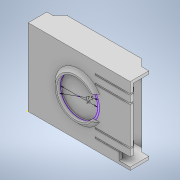
# Autodesk Inventor part: ButtonBatteryHolder
Saved by Autodesk Inventor 2022 (Build 260153000, 153)
## iProperties
Created: 2022-08-02
Part Number: ButtonBatteryHolder
Material: Generic
Document SubType Name: Modeling
Designer: sgioj
Density: 1 g/cm^3
Appearance: Default
Author: sgioj
Autodesk Inventor part; units mm, degrees
ref_plane "YZ Plane" through (0, 0, 0) normal (1, 0, 0) x (0, 1, 0)
ref_plane "XZ Plane" through (0, 0, 0) normal (0, 1, 0) x (-1, 0, 0)
ref_plane "XY Plane" through (0, 0, 0) normal (0, 0, 1) x (1, 0, 0)
sketch "Sketch1" plane through (0, 0, 0) normal (0, 0, 1) x (1, 0, 0)
  line L0 (0, 0) -> (44, 0)
  line L1 (44, 0) -> (44, 33)
  line L2 (44, 33) -> (0, 33)
  line L3 (0, 33) -> (0, 0)
  line L4 (2, 1.5) -> (44, 1.5)
  line L5 (44, 1.5) -> (44, 31.5)
  line L6 (44, 31.5) -> (2, 31.5)
  line L7 (2, 31.5) -> (2, 1.5)
  dimension "d0" = 44
  dimension "d1" = 33
  dimension "d2" = 42
  dimension "d3" = 30
  dimension "d4" = 2
  dimension "d5" = 0
  dimension "d6" = 1.5
  constraints: 16 end point, 4 parallel, 2 horizontal, 2 perpendicular
  measures "d0" distance of L2.end L1.end
  measures "d1" distance of L1.end L0.end
  measures "d2" distance of L6.end L5.end
  measures "d3" distance of L5.end L4.end
  measures "d4" distance between parallel lines of L7 L3
  measures "d5" distance between parallel lines of L1 L5
  measures "d6" distance between parallel lines of L4 L0
extrude "Extrusion1" add sketch "Sketch1" along normal blind 11
shell "Shell1" thickness 1.25 removed faces 1 at (44, 11, 3.6667)
sketch "Sketch2" plane through (0, 0, 11) normal (0, 0, 1) x (1, 0, 0)
  circle A0 centre (22, 16.5) radius 8
  circle A1 centre (22, 16.5) radius 8.75
  point P0 (0, 0)
  dimension "d10" = 16
  dimension "d11" = 17.5
  constraints: 2 centre point, 1 coincident
  measures "d10" diameter of A0
  measures "d11" diameter of A1
extrude "Extrusion2" add sketch "Sketch2" along normal blind 1.5
sketch "Sketch3" plane through (22, 16.5, 11) normal (0, 0, 1) x (1, 0, 0)
  line L0 (1.47, 5.1769) -> (11.6334, 5.1769)
  line L1 (11.6334, 5.1769) -> (11.6334, -5.2059)
  line L2 (11.6334, -5.2059) -> (1.47, -5.2059)
  line L3 (1.47, -5.2059) -> (1.47, 5.1769)
  line L4 (1.47, 5.1769) -> (11.6334, -5.2059) construction
  line L5 (11.6334, 5.1769) -> (1.47, -5.2059) construction
  point P0 (-22, -16.5)
  point P1 (6.5517, -0.0145)
  constraints: 12 end point, 2 midpoint, 2 parallel, 1 horizontal, 1 perpendicular
extrude "Extrusion3" cut sketch "Sketch2" against normal blind 0.6 contours A0
sketch "Sketch4" plane through (0, 0, 0) normal (0, 0, -1) x (-1, 0, 0)
  circle A0 centre (-22, 16.5) radius 8.7
  line L0 (-44, 33) -> (0, 33) projected
  line L1 (0, 33) -> (0, 0) projected
  dimension "d16" = 17.4
  dimension "d22" = 16.5
  dimension "d23" = 22
  constraints: 1 centre point
  measures "d16" diameter of A0
  measures "d22" distance from line of L0 A0.centre
  measures "d23" distance from line of L1 A0.centre
extrude "Extrusion4" cut sketch "Sketch4" against normal blind 0.6
chamfer "Chamfer1" distance 1.5 angle 45 1 edges at (13.25, 16.5, 11)
extrude "Extrusion5" cut sketch "Sketch3" along normal blind 2
sketch "Sketch5" plane through (0, 33, 0) normal (0, 1, 0) x (1, 0, 0)
  line L0 (0, 0) -> (3, 0)
  line L1 (3, 0) -> (3, -3)
  line L2 (3, -3) -> (0, -3)
  line L3 (0, -3) -> (0, 0)
  line L4 (0, 0) -> (44, 0) projected
  line L5 (44, 0) -> (41, 0)
  line L6 (41, 0) -> (41, -3)
  line L7 (41, -3) -> (44, -3)
  line L8 (44, -3) -> (44, 0)
  dimension "d26" = 3
  dimension "d27" = 3
  dimension "d28" = 3
  dimension "d29" = 3
  constraints: 16 end point, 4 parallel, 2 horizontal, 2 perpendicular
  measures "d26" distance of L1.end L2.end
  measures "d27" distance of L0.end L1.end
  measures "d28" distance of L7.end L6.end
  measures "d29" distance of L6.end L5.end
extrude "Extrusion6" cut sketch "Sketch5" against normal through all
sketch "Sketch6" plane through (0, 0, 11) normal (-1, 0, 0) x (0, 0, 1)
  line L0 (0, 0) -> (0, 33) projected
  line L1 (-11, 33) -> (-11, 0) projected
  line L2 (0, 0) -> (-11, 0)
  line L3 (-11, 0) -> (-11, 33)
  line L4 (-11, 33) -> (0, 33)
  line L5 (0, 33) -> (0, 0)
  constraints: 8 end point, 2 parallel, 1 horizontal, 1 perpendicular
extrude "Extrusion7" cut sketch "Sketch6" against normal blind 0.25
chamfer "Chamfer2" distance 3 angle 45 2 edges at (3, 16.5, 0) (41, 16.5, 0)
sketch "Sketch7" plane through (0, 0, 11) normal (0, 0, 1) x (1, 0, 0)
  line L0 (44, 1.25) -> (44, 31.75) projected
  line L1 (44, 28) -> (29, 28)
  line L2 (29, 28) -> (29, 25)
  line L3 (29, 25) -> (44, 25)
  line L4 (44, 25) -> (44, 28)
  line L5 (44, 33) -> (0.25, 33) projected
  line L6 (44, 28.5) -> (29, 28.5)
  line L7 (29, 28.5) -> (29, 24.5)
  line L8 (29, 24.5) -> (44, 24.5)
  line L9 (44, 24.5) -> (44, 28.5)
  point P0 (0, 0)
  dimension "d37" = 15
  dimension "d38" = 3
  dimension "d39" = 5
  dimension "d40" = 4
  constraints: 16 end point, 4 parallel, 2 horizontal, 2 perpendicular, 2 point on line
  measures "d37" distance of L3.end L2.end
  measures "d38" distance of L2.end L1.end
  measures "d39" distance between parallel lines of L5 L1
  measures "d40" distance of L7.end L6.end
extrude "Extrusion8" cut sketch "Sketch7" against normal blind 1.5 contours L8 L7 L3 L0 | L1 L7 L6 L0
sketch "Sketch8" plane through (44, 1.25, 9.75) normal (0, 0, -1) x (-1, 0, 0)
  line L0 (0, 26.75) -> (15, 26.75) projected
  line L1 (0, 23.75) -> (15, 23.75) projected
  line L2 (0, 26.75) -> (4.5, 26.75)
  line L3 (4.5, 26.75) -> (4.5, 23.75)
  line L4 (4.5, 23.75) -> (0, 23.75)
  line L5 (0, 23.75) -> (0, 26.75)
  point P0 (44, -1.25)
  point P1 (4.5, 26.75)
  dimension "d43" = 4.5
  constraints: 8 end point, 2 parallel, 1 horizontal, 1 perpendicular, 1 point on line
  measures "d43" distance of L3.end L4.end
extrude "Extrusion9" add sketch "Sketch8" along normal blind 2.5
chamfer "Chamfer3" distance 2.25 angle 45 2 edges at (44, 26.5, 7.25) (39.5, 26.5, 7.25)
pattern_linear "Rectangular Pattern1" count 2 spacing 20 along (0, -1, 0) of "Extrusion9", "Chamfer3", "Extrusion8"
sketch "Sketch9" plane through (0, 0, 11) normal (0, 0, 1) x (1, 0, 0)
  line L0 (44, 4.5) -> (29, 4.5) projected
  line L1 (4.75, 1.25) -> (39.25, 1.25) projected
  line L2 (44, 4.5) -> (39.25, 4.5)
  line L3 (39.25, 4.5) -> (39.25, 1.25)
  line L4 (39.25, 1.25) -> (44, 1.25)
  line L5 (44, 1.25) -> (44, 4.5)
  point P0 (0, 0)
  constraints: 8 end point, 2 parallel, 1 horizontal, 1 perpendicular
extrude "Extrusion10" cut sketch "Sketch9" against normal blind 2.5
body "Solid1"
